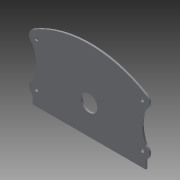
# Autodesk Inventor part: Berring plate M
Saved by Autodesk Inventor 2014 SP1 (Build 180222100, 222)
## iProperties
Created: 2014-01-13
Part Number: Berring plate M
Material: Generic
Document SubType Name: Sheet Metal
Designer: noah
Density: 1 g/cm^3
Sheet Metal Rule: Default
Appearance: Default
Author: noah
Autodesk Inventor part; units mm, degrees
ref_plane "YZ Plane" through (0, 0, 0) normal (1, 0, 0) x (0, 1, 0)
ref_plane "XZ Plane" through (0, 0, 0) normal (0, 1, 0) x (-1, 0, 0)
ref_plane "XY Plane" through (0, 0, 0) normal (0, 0, 1) x (1, 0, 0)
sketch "Sketch1" plane through (0, 0, 0) normal (0, 0, 1) x (1, 0, 0)
  line L0 (0, 0) -> (196.85, 0)
  line L1 (196.85, 0) -> (196.85, 139.7)
  line L2 (196.85, 139.7) -> (0, 139.7)
  line L3 (0, 139.7) -> (0, 0)
  circle A0 centre (98.425, 50.8) radius 14.2875
  dimension "d0" = 196.85
  dimension "d1" = 139.7
  dimension "d2" = 28.575
  dimension "d3" = 50.8
  dimension "d4" = 98.425
  measures "d0" distance of L2.end L1.end
  measures "d1" distance between parallel lines of L2 L0
  measures "d2" diameter of A0
  measures "d3" distance from line of A0.centre L0
  measures "d4" distance from line of A0.centre L1
extrude "Plate1" add sketch "Sketch1" along normal blind 3.048
sketch "Sketch2" plane through (0, 0, 0) normal (0, 0, -1) x (-1, 0, 0)
  circle A0 centre (-190.5, 101.6) radius 3.175 projected
  circle A1 centre (-190.5, 25.4) radius 3.175 projected
  circle A2 centre (-6.35, 101.6) radius 3.175 projected
  circle A3 centre (-6.35, 25.4) radius 3.175 projected
  arc A4 (-19.05, 50.8) -> (-177.8, 50.8) centre (-98.425, 50.8) ccw projected
sketch "Sketch3" plane through (0, 0, 0) normal (0, 0, -1) x (-1, 0, 0)
  line L0 (0, 0) -> (-196.85, 0)
  line L1 (0, 139.7) -> (0, 0)
  line L2 (-196.85, 139.7) -> (0, 139.7)
  line L3 (-196.85, 0) -> (-196.85, 139.7)
  circle A0 centre (-98.425, 50.8) radius 14.2875
  line L4 (0, 0) -> (-196.85, 0)
  line L5 (0, 139.7) -> (0, 0)
  line L6 (-196.85, 139.7) -> (0, 139.7)
  line L7 (-196.85, 0) -> (-196.85, 139.7)
  circle A1 centre (-6.35, 101.6) radius 3.175
  circle A2 centre (-6.35, 25.4) radius 3.175
  circle A3 centre (-190.5, 101.6) radius 3.175
  circle A4 centre (-190.5, 25.4) radius 3.175
  arc A5 (-19.05, 50.8) -> (-177.8, 50.8) centre (-98.425, 50.8) ccw
  circle A6 centre (-190.5, 101.6) radius 12.7
  circle A7 centre (-190.5, 25.4) radius 12.7
  circle A8 centre (-6.35, 25.4) radius 12.7
  circle A9 centre (-6.35, 101.6) radius 12.7
  arc A10 (0, 112.5985) -> (-196.85, 112.5985) centre (-98.425, -52.5768) ccw
  dimension "d6" = 25.4
  measures "d6" diameter of A8
sheet face with bend "Face2" sketch "Sketch3" thickness 3.048 toward (0, 0, 1) bend radius 3.048 relief straight relief width 3.048 relief depth 1.524 contours A8 L1 | L1 A8 | A7 L3 | L3 A7 | A9 L1 | L1 A9 | A6 L3 | L3 A6 | A10 L2 L1 | L3 L2 A10
bend "Bend1"
sketch "Sketch4" plane through (0, 0, 0) normal (0, 0, -1) x (-1, 0, 0)
  line L0 (-196.85, 36.3985) -> (-196.85, 90.6015) projected
  arc A0 (-196.85, 36.3985) -> (-196.85, 14.4015) centre (-190.5, 25.4) ccw projected
  line L1 (-196.85, 0) -> (-196.85, 14.4015) projected
  line L2 (0, 0) -> (-196.85, 0) projected
  line L3 (0, 14.4015) -> (0, 0) projected
  arc A1 (0, 14.4015) -> (0, 36.3985) centre (-6.35, 25.4) ccw projected
  line L4 (0, 90.6015) -> (0, 36.3985) projected
  arc A2 (0, 90.6015) -> (0, 112.5985) centre (-6.35, 101.6) ccw projected
  line L5 (0, 139.7) -> (0, 112.5985) projected
  line L6 (-196.85, 139.7) -> (0, 139.7) projected
  line L7 (-196.85, 112.5985) -> (-196.85, 139.7) projected
  arc A3 (-196.85, 112.5985) -> (-196.85, 90.6015) centre (-190.5, 101.6) ccw projected
  arc A4 (0, 112.5985) -> (-196.85, 112.5985) centre (-98.425, -52.5768) ccw
  arc A5 (-196.85, 36.3985) -> (-196.85, 90.6015) centre (-250.6784, 63.5) ccw
  arc A6 (0, 90.6015) -> (0, 36.3985) centre (54.4604, 63.5) ccw
  constraints: 6 point on circle, 3 centre point, 1 tangent
extrude "Cut1" cut sketch "Sketch4" against normal blind 3.048 contours L0 A5 | L7 L6 A4 | L6 L5 A4 | L4 A6
extrude "Cut2" cut sketch "Sketch2" against normal blind 3.048
equation "\"d12\" = Thickness"
equation "\"d14\" = Thickness"
equation "\"d7\" = BendRadius"
equation "\"d8\" = BendReliefWidth"
equation "\"d10\" = MinimumRemnant"
equation "\"d9\" = BendReliefDepth"
equation "\"d11\" = BendRadius"
equation "\"BendRadius\" = Thickness"
equation "\"BendReliefWidth\" = Thickness"
equation "\"BendReliefDepth\" = 0.5 * Thickness"
equation "\"CornerReliefSize\" = 4 * Thickness"
equation "\"MinimumRemnant\" = 2 * Thickness"
equation "\"TransitionRadius\" = BendRadius"
equation "\"JacobiRadiusSize\" = BendRadius"
equation "\"GapSize\" = Thickness"
equation "\"d5\" = BendRadius"
equation "\"Thickness\" = 3.048"
body "Solid1"
